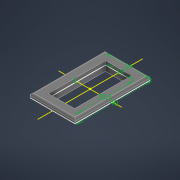
# Autodesk Inventor part: Ramecek
Saved by Autodesk Inventor 2022 (Build 260153000, 153)
## iProperties
Created: 2021-05-08
Part Number: Ramecek
Material: Generic
Document SubType Name: Modeling
Designer: jodyn
Density: 1 g/cm^3
Appearance: Gray
Author: jodyn
## iProperties of the stored document Ramecek_3DPrint.ipt
Created: 2021-05-08
Part Number: Ramecek_3DPrint
Material: Generic
Document SubType Name: Modeling
Designer: jodyn
Density: 1 g/cm^3
Appearance: Default
Author: jodyn
Autodesk Inventor part; units mm, degrees
ref_plane "YZ Plane" through (0, 0, 0) normal (1, 0, 0) x (0, 1, 0)
ref_plane "XZ Plane" through (0, 0, 0) normal (0, 1, 0) x (-1, 0, 0)
ref_plane "XY Plane" through (0, 0, 0) normal (0, 0, 1) x (1, 0, 0)
sketch "Sketch1" plane through (0, 0, 0) normal (0, 1, 0) x (-1, 0, 0)
  line L0 (0, -28) -> (0, 28) projected
  line L1 (16.8, 0) -> (-16.8, 0) projected
  line L2 (7, 15.25) -> (-7, 15.25)
  line L3 (-7, 15.25) -> (-7, -15.25)
  line L4 (-7, -15.25) -> (7, -15.25)
  line L5 (7, -15.25) -> (7, 15.25)
  line L6 (9, 17.25) -> (-9, 17.25)
  line L7 (-9, 17.25) -> (-9, -17.25)
  line L8 (-9, -17.25) -> (9, -17.25)
  line L9 (9, -17.25) -> (9, 17.25)
  line L10 (12, 20) -> (-12, 20)
  line L11 (-12, 20) -> (-12, -20)
  line L12 (-12, -20) -> (12, -20)
  line L13 (12, -20) -> (12, 20)
  point P0 (0, 0)
  dimension "d0" = 14
  dimension "d1" = 30.5
  dimension "d2" = 2
  dimension "d3" = 24
  dimension "d4" = 40
  constraints: 24 end point, 6 parallel, 3 perpendicular, 2 horizontal, 7 other
  measures "d0" distance of L4.end L3.end
  measures "d1" distance of L3.end L2.end
  measures "d2" distance between parallel lines of L5 L9
  measures "d3" distance of L12.end L11.end
  measures "d4" distance of L11.end L10.end
extrude "Extrusion1" add sketch "Sketch1" against normal blind 3 contours L8 L7 L1 L3 L4 L0 | L0 L4 L5 L1 L9 L8 | L7 L6 L0 L2 L3 L1 | L1 L5 L2 L0 L6 L9
extrude "Extrusion2" add sketch "Sketch1" along normal blind 2 contours L12 L11 L1 L7 L8 L0 | L0 L8 L9 L1 L13 L12 | L8 L7 L1 L3 L4 L0 | L0 L4 L5 L1 L9 L8 | L11 L10 L0 L6 L7 L1 | L1 L9 L6 L0 L10 L13 | L7 L6 L0 L2 L3 L1 | L1 L5 L2 L0 L6 L9
fillet "Fillet1" radius 1 4 edges at (-12, 2, 0) (0, 2, -20) (12, 2, 0) (0, 2, 20)
body "Solid1"
